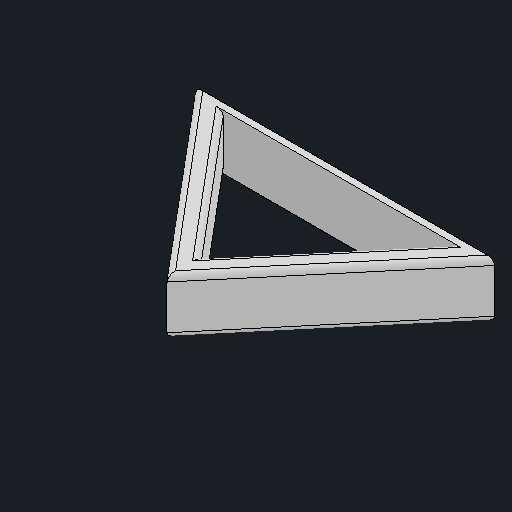
# Autodesk Inventor part: test-triangle-overhang
Saved by Autodesk Inventor 2026 (Build 300175050, 175E)
## iProperties
Created: 2026-01-09
Part Number: test-triangle-overhang
Material: Generic
Document SubType Name: Modeling
Designer: kuzmin
Density: 1 g/cm^3
Appearance: Default
Author: kuzmin
Autodesk Inventor part; units mm, degrees
ref_plane "YZ Plane" through (0, 0, 0) normal (1, 0, 0) x (0, 1, 0)
ref_plane "XZ Plane" through (0, 0, 0) normal (0, 1, 0) x (-1, 0, 0)
ref_plane "XY Plane" through (0, 0, 0) normal (0, 0, 1) x (1, 0, 0)
sketch "Sketch1" plane through (0, 0, 0) normal (0, 1, 0) x (-1, 0, 0)
  line L0 (-20.9775, 0) -> (0, 25)
  line L1 (0, 25) -> (20.9775, 0)
  line L2 (20.9775, 0) -> (-20.9775, 0)
  line L3 (0, 25) -> (0, 0) construction
  line L4 (0, 31.2229) -> (-29.5555, -4)
  line L5 (-29.5555, -4) -> (29.5555, -4)
  line L6 (29.5555, -4) -> (0, 31.2229)
  line L7 (27.206, -1.2) -> (-27.206, -1.2)
  dimension "d0" = 40
  dimension "d1" = 25
  dimension "d2" = 4
  dimension "d6" = 1.2
  constraints: 16 end point, 2 horizontal, 2 point on line, 1 equal length, 1 midpoint, 1 vertical, 1 vertical alignment, 2 other
  measures "d0" angle of L1 L3
  measures "d1" distance of L0.end L3.end
  measures "d2" distance between parallel lines of L6 L1
  measures "d6" distance between parallel lines of L7 L2
extrude "Extrusion1" add sketch "Sketch1" along normal blind 10 contours L6 L7 L4
fillet "Fillet1" radius 1 8 edges at (10.4887, 10, 12.5) (-10.4887, 10, 12.5) (-13.603, 0, 15.0114) (-10.4887, 0, 12.5) (-13.603, 10, 15.0114) (10.4887, 0, 12.5) (13.603, 0, 15.0114) (13.603, 10, 15.0114)
body "Solid1"
